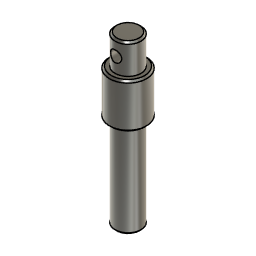
Pos31 (Autodesk Fusion 360 design; units mm, degrees)
Autodesk Fusion 360 part; units mm, degrees
sketch "Boceto1" plane through (0, 0, 0) normal (0, 0, 1) x (1, 0, 0)
  line L0 (0, 43) -> (3, 43)
  line L1 (3, 43) -> (3.5, 42.5)
  line L2 (3.5, 42.5) -> (3.5, 35)
  line L3 (3.5, 35) -> (4.5, 35)
  line L4 (4.5, 35) -> (5, 34.5)
  line L5 (5, 34.5) -> (5, 20.5)
  line L6 (5, 20.5) -> (4.5, 20)
  line L7 (4.5, 20) -> (3.5, 20)
  line L8 (3.5, 20) -> (3.5, 0.5)
  line L9 (3.5, 0.5) -> (3, 0)
  line L10 (3, 0) -> (0, 0)
  line L11 (0, 0) -> (0, 43)
  dimension "d2" = 45
  dimension "d3" = 0.5
  dimension "d4" = 0.5
  dimension "d5" = 0.5
  dimension "d6" = 0.5
  dimension "d7" = 3
  dimension "d8" = 8
  dimension "d9" = 15
  dimension "d10" = 43
  dimension "d12" = 5
  constraint horizontal L0
  constraint perpendicular L0 L2
  constraint perpendicular L2 L3
  constraint parallel L1 L4
  constraint perpendicular L3 L5
  constraint perpendicular L4 L6
  constraint perpendicular L5 L7
  constraint perpendicular L7 L8
  constraint parallel L6 L9
  constraint perpendicular L8 L10
  constraint perpendicular L0 L11
  constraint vertical L2.end L7.end
  constraint coincident L10.end L11.start
  measures "d2" angle of L1 L2
  measures "d3" distance of L0 L1.end
  measures "d4" vertical distance of L3.end L4.end
  measures "d5" vertical distance of L5.end L6.end
  measures "d6" vertical distance of L8.end L9.end
  measures "d7" distance of L0.start L0.end
  measures "d8" distance of L0 L3
  measures "d9" distance of L3 L7
  measures "d10" distance of L0.start L10.end
  measures "d12" distance of L5 L11
sketch "Boceto2" plane through (0, 0, 0) normal (0, 1, 0) x (1, 0, 0)
  line L0 (-3, 0) -> (0, 0)
  line L1 (-4.5, -25) -> (-3.5, -25)
  line L2 (-3.5, -44.5) -> (-3.5, -37)
  line L3 (0, -45) -> (-3, -45)
  line L4 (-5, -36.5) -> (-5, -25.5)
  line L5 (-3.5, -37) -> (-4.5, -37)
  line L6 (-4.5, -37) -> (-5, -36.5)
  line L7 (-5, -25.5) -> (-4.5, -25)
  line L8 (0, 0) -> (0, -45)
  line L9 (-3, -45) -> (-3.5, -44.5)
  line L10 (-3.5, -25) -> (-3.5, -0.5)
  line L11 (-3.5, -0.5) -> (-3, 0)
  dimension "d13" = 45
  dimension "d14" = 0.5
  dimension "d18" = 3
  dimension "d19" = 8
  dimension "d20" = 12
  dimension "d21" = 45
  dimension "d22" = 5
  dimension "d28" = 0.5
  dimension "d29" = 0.5
  constraint perpendicular L2 L3
  constraint perpendicular L2 L5
  constraint parallel L6 L9
  constraint perpendicular L4 L5
  constraint perpendicular L6 L7
  constraint perpendicular L1 L4
  constraint perpendicular L1 L10
  constraint parallel L7 L11
  constraint perpendicular L0 L10
  constraint perpendicular L3 L8
  constraint coincident L0.end L8.start
  measures "d13" angle of L2 L9
  measures "d14" distance of L2.start L3
  measures "d18" distance of L3.end L3.start
  measures "d19" distance of L3 L5
  measures "d20" distance of L1 L5
  measures "d21" distance of L3.start L0.end
  measures "d22" distance of L4 L8
  measures "d28" vertical distance of L4.start L5.end
  measures "d29" vertical distance of L4.end L1.start
revolve "Revolución1" add sketch "Boceto2" angle 360 about axis through (0, 0, 0) along (0, 0, 1)
sketch "Boceto3" plane through (0, 0, 0) normal (0, 1, 0) x (1, 0, 0)
  circle A0 centre (0, -41) radius 1.5
  line L0 (3, -45) -> (-3, -45)
  dimension "d24" = 4
  dimension "d25" = 3
  constraint vertical origin A0.centre
  measures "d24" distance of A0.centre L0
  measures "d25" diameter of A0
extrude "Extruir1" cut sketch "Boceto3" along normal mid plane 10
